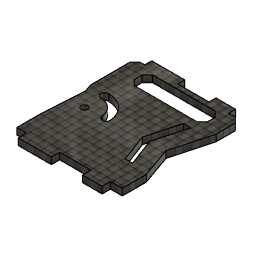
fpv_camera_mount (Autodesk Fusion 360 design; units mm, degrees)
Autodesk Fusion 360 part; units mm, degrees
sketch "Sketch1" plane through (0, 0, 0) normal (0, 1, 0) x (1, 0, 0)
  line L0 (0, 0) -> (0, 38) construction
  line L1 (-64.8988, -2.8025) -> (-29.1208, -2.8025) construction
  line L2 (-56.5735, -2.8025) -> (-56.5735, -0.3025)
  line L3 (-46.6235, -0.3025) -> (-46.6235, -2.8025)
  line L4 (-37.2465, -2.8025) -> (-37.2465, -0.3025)
  line L5 (-46.6235, -0.3025) -> (-37.2465, -0.3025)
  line L6 (-56.5735, -0.3025) -> (-59.486, -0.3025)
  line L7 (-56.5735, -2.8025) -> (-46.6235, -2.8025)
  line L8 (-37.2465, -2.8025) -> (-31.3465, -2.8025)
  line L9 (-31.3465, -2.8025) -> (-31.3465, -0.3025)
  line L10 (-31.3465, -0.3025) -> (-27.7965, -0.3025)
  line L11 (-64.8988, -2.8025) -> (-64.8988, 12.2374) construction
  line L12 (-69.2513, 0.6975) -> (-69.2513, 34.6975) construction
  line L13 (-69.2513, 17.6975) -> (-81, 17.6975) construction
  line L14 (-46.6235, 35.1975) -> (-46.6235, 37.3057)
  line L15 (-56.5735, 37.3057) -> (-56.5735, 35.1975)
  line L16 (-56.5735, 37.3057) -> (-46.6235, 37.3057)
  line L17 (-46.6235, 35.1975) -> (-37.2465, 35.1975)
  line L18 (-37.2465, 37.2981) -> (-31.3465, 37.2981)
  line L19 (-37.2465, 37.2981) -> (-37.2465, 35.1975)
  line L20 (-31.3465, 37.2981) -> (-31.3465, 35.1975)
  line L21 (-29.2965, 35.1975) -> (-31.3465, 35.1975)
  line L22 (-52.3267, 32.7382) -> (-34.3267, 32.7382)
  line L23 (-33.3267, 31.7382) -> (-33.3267, 30.2382)
  line L24 (-34.3267, 29.2382) -> (-52.3267, 29.2382)
  line L25 (-53.3267, 30.2382) -> (-53.3267, 31.7382)
  line L26 (-52.3267, 32.7382) -> (-53.3267, 31.7382)
  line L27 (-53.3267, 30.2382) -> (-52.3267, 29.2382)
  line L28 (-33.3267, 31.7382) -> (-34.3267, 32.7382)
  line L29 (-33.3267, 30.2382) -> (-34.3267, 29.2382)
  line L30 (-56.5735, 35.1975) -> (-57.986, 35.1975)
  line L31 (-57.986, 35.1975) -> (-59.486, 33.6975)
  line L32 (-29.2965, 35.1975) -> (-27.7965, 33.6975)
  line L33 (-27.7965, 27.8812) -> (-31, 16)
  line L34 (-31, 16) -> (-27.7965, 6.8866)
  line L35 (-27.7965, -0.3025) -> (-27.7965, 6.8866)
  line L36 (-27.7965, 27.8812) -> (-27.7965, 33.6975)
  line L37 (-59.486, 21.8801) -> (-58.6446, 19.4865)
  line L38 (-58.6446, 19.4865) -> (-59.486, 6.8454)
  line L39 (-59.486, 33.6975) -> (-59.486, 21.8801)
  line L40 (-59.486, 6.8454) -> (-59.486, -0.3025)
  line L41 (-33.2612, 25.74) -> (-35.8874, 16)
  line L42 (-35.8874, 16) -> (-32.781, 7.7708)
  line L43 (-32.781, 7.7708) -> (-34.9986, 7.7708)
  line L44 (-34.9986, 7.7708) -> (-38.1062, 16.003)
  line L45 (-38.1062, 16.003) -> (-35.4808, 25.74)
  line L46 (-35.4808, 25.74) -> (-33.2612, 25.74)
  circle A0 centre (-54.5087, 15.0402) radius 1
  line L47 (-65.4941, 32.6975) -> (-65.4941, 3) construction
  line L48 (-65.4941, 17.8488) -> (-22, 17.8488) construction
  circle A1 centre (-54.5087, 15.0402) radius 6.0725 construction
  circle A2 centre (-54.5087, 15.0402) radius 12 construction
  circle A3 centre (-54.5087, 15.0402) radius 8 construction
  arc A4 (-47.3058, 15.6327) -> (-54.4948, 22.2674) centre (-54.5087, 15.0402) ccw
  arc A5 (-49.6075, 15.4433) -> (-47.3058, 15.6327) centre (-48.4567, 15.538) ccw
  arc A6 (-49.6075, 15.4433) -> (-54.4992, 19.9579) centre (-54.5087, 15.0402) ccw
  arc A7 (-54.4948, 22.2674) -> (-54.4992, 19.9579) centre (-54.497, 21.1127) ccw
  arc A8 (-48.4567, 15.538) -> (-54.497, 21.1127) centre (-54.5087, 15.0402) ccw construction
  line L49 (-32.3267, 32.1524) -> (-33.9125, 33.7382)
  line L50 (-52.7409, 33.7382) -> (-33.9125, 33.7382)
  line L51 (-52.7409, 33.7382) -> (-54.3267, 32.1524)
  line L52 (-54.3267, 29.824) -> (-54.3267, 32.1524)
  line L53 (-54.3267, 29.824) -> (-52.7409, 28.2382)
  line L54 (-33.9125, 28.2382) -> (-52.7409, 28.2382)
  line L55 (-32.3267, 29.824) -> (-33.9125, 28.2382)
  line L56 (-32.3267, 32.1524) -> (-32.3267, 29.824)
  point P0 (-27.7965, 35.1975)
  point P1 (-64.8988, 34.6975)
  point P2 (-53.3267, 32.7382)
  point P3 (-33.3267, 32.7382)
  point P4 (-53.3267, 29.2382)
  point P5 (-33.3267, 29.2382)
  point P6 (-59.486, 35.1975)
  dimension "d14" = 35.778
  dimension "d18" = 9.95
  dimension "d19" = 9.377
  dimension "d21" = 5.9
  dimension "d22" = 2.5
  dimension "d23" = 3.55
  dimension "d25" = 2.5
  dimension "d26" = 2.5
  dimension "d27" = 20
  dimension "d28" = 3.5
  dimension "d29" = 1
  dimension "d30" = 1
  dimension "d31" = 1
  dimension "d32" = 1
  dimension "d33" = 1
  dimension "d35" = 1
  dimension "d40" = 1
  dimension "d41" = 1
  dimension "d42" = 1.5
  dimension "d43" = 1.5
  dimension "d44" = 1.5
  dimension "d45" = 1.5
  dimension "d56" = 2
  dimension "d58" = 24
  dimension "d59" = 16
  dimension "d61" = 1
  constraint coincident L0.start origin
  constraint vertical L0
  constraint horizontal L1
  constraint coincident L1 L2.start
  constraint coincident L1 L3.end
  constraint perpendicular L4 L8
  constraint coincident L1 L8.end
  constraint perpendicular L1 L9
  constraint perpendicular L9 L10
  constraint parallel L1 L6
  constraint parallel L1 L5
  constraint perpendicular L1 L11
  constraint parallel L2 L11
  constraint parallel L3 L11
  constraint parallel L4 L11
  constraint parallel L11 L35
  constraint perpendicular L1 L12
  constraint midpoint L12 L13.start
  constraint perpendicular L12 L13
  constraint perpendicular L20 L21
  constraint horizontal L22
  constraint vertical L23
  constraint horizontal L24
  constraint vertical L25
  constraint coincident P2 L22
  constraint coincident P2 L25
  constraint coincident P4 L25
  constraint coincident P4 L24
  constraint coincident P3 L23
  constraint coincident P3 L22
  constraint coincident L23 P5
  constraint coincident L24 P5
  constraint perpendicular L6 L39
  constraint perpendicular L30 L39
  constraint coincident L30 P6
  constraint coincident P6 L39
  constraint coincident P0 L21
  constraint coincident P0 L35
  constraint coincident L33.start L35
  constraint collinear L35 L36
  constraint parallel L34 L37
  constraint coincident L38.end L39
  constraint collinear L39 L40
  constraint parallel L33 L41
  constraint horizontal L43
  constraint parallel L42 L44
  constraint parallel L43 L46
  constraint perpendicular L30 L47
  constraint midpoint L47 L48.start
  constraint perpendicular L47 L48
  constraint concentric A0 A1
  constraint concentric A0 A2
  constraint concentric A1 A3
  constraint tangent A4 A5
  constraint tangent A5 A6
  constraint tangent A6 A7
  constraint tangent A4 A7
  constraint coincident A0.centre A1.centre
  constraint coincident A1 A7.centre
  constraint coincident L37.end A1
  measures "d14" distance of L1.start L1.end
  measures "d18" horizontal distance of L2.end L3.start
  measures "d19" distance of L3.end L4.start
  measures "d21" distance of L4.start L8.end
  measures "d22" distance of L8.end L9.end
  measures "d23" distance of L9.end L10.end
  measures "d25" distance of L2.start L2.end
  measures "d26" distance of L3.start L3.end
  measures "d27" distance of P2 P3
  measures "d28" distance of P2 P4
  measures "d29" distance of P2 L22.start
  measures "d30" distance of P2 L25.end
  measures "d31" distance of P4 L25.start
  measures "d32" distance of P4 L24.end
  measures "d33" distance of P3 L23.start
  measures "d35" distance of P3 L22.end
  measures "d40" distance of L23.end P5
  measures "d41" distance of L24.start P5
  measures "d42" distance of L30.end P6
  measures "d43" distance of L31.end P6
  measures "d44" distance of P0 L21.start
  measures "d45" distance of P0 L32.end
  measures "d56" diameter of A0
  measures "d58" diameter of A2
  measures "d59" diameter of A3
  measures "d61" distance of L28
extrude "Extrude1" add sketch "Sketch1" along normal blind 2 contours L2 L3 L4 L5 L6 L7 L8 L9 L10 L14 L15 L16 L17 L18 L19 L20 L21 L30 L31 L32 L33 L34 L35 L36 L37 L38 L39 L40
equation "d30 = d29"
equation "d32 = d31"
equation "d35 = d33"
equation "d41 = d40"
equation "d43 = d42"
equation "d45 = d44"
